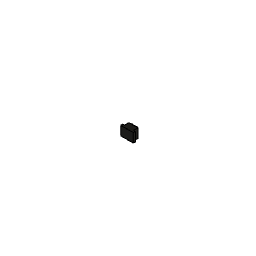
Taste7_v56 (Autodesk Fusion 360 design; units mm, degrees)
Autodesk Fusion 360 part; units mm, degrees
sketch "Skizze1" plane through (0, 0, 59.536) normal (0, 0, -1) x (1, 0, 0)
  line L0 (54.288, -85.97) -> (62.288, -85.97)
  line L1 (62.288, -85.97) -> (62.288, -82.97)
  line L2 (62.288, -82.97) -> (54.288, -82.97)
  line L3 (54.288, -82.97) -> (54.288, -85.97)
  line L4 (63.688, -82.82) -> (62.188, -82.82)
  line L5 (62.188, -82.82) -> (62.188, -86.47)
  line L6 (62.188, -86.47) -> (54.588, -86.47)
  line L7 (54.588, -86.47) -> (54.588, -82.82)
  line L8 (54.588, -82.82) -> (53.088, -82.82)
  line L9 (53.088, -82.82) -> (53.088, -81.07)
  line L10 (53.088, -81.07) -> (63.688, -81.07)
  line L11 (63.688, -81.07) -> (63.688, -82.82)
  line L12 (-67.1, -82.97) -> (67.1, -82.97)
  line L13 (56.538, -80.97) -> (60.038, -80.97)
  line L14 (50.288, -82.97) -> (50.288, -85.97)
  point P0 (54.288, -85.97)
  point P1 (50.288, -85.97)
  dimension "d139" = 1.5
  dimension "d140" = 1.5
  dimension "d1183" = 1.75
  dimension "d1184" = 3.65
  dimension "d1185" = 7.6
  constraint horizontal L4
  constraint perpendicular L0 L5
  constraint perpendicular L5 L6
  constraint perpendicular L0 L7
  constraint perpendicular L7 L8
  constraint perpendicular L0 L9
  constraint perpendicular L7 L10
  constraint perpendicular L10 L11
  constraint horizontal L4.end L7.end
  measures "d139" distance of L7.end L8.end
  measures "d140" distance of L4.start L4.end
  measures "d1183" distance of L8.end L9.end
  measures "d1184" distance of L6.end L7.end
  measures "d1185" distance of L5.end L6.end
extrude "Extrusion1" add sketch "Skizze1" along normal blind 7.6 contours L0 L2 L5 L7 L12 | L0 L5 L6 L7 | L2 L4 L5 L7 L8 L9 L10 L11 L12
sketch "Skizze2" plane through (0, 86.47, 0) normal (0, 1, 0) x (-1, 0, 0)
  line L0 (-54.588, 59.536) -> (-62.188, 59.536)
  line L1 (-62.188, 59.536) -> (-62.188, 51.936)
  line L2 (-62.188, 51.936) -> (-54.588, 51.936)
  line L3 (-54.588, 51.936) -> (-54.588, 59.536)
  line L4 (-60.8264, 52.636) -> (-55.9496, 52.636) construction
  line L5 (-55.9496, 52.636) -> (-55.9496, 61.236) construction
  line L6 (-55.9496, 61.236) -> (-60.8264, 61.236) construction
  line L7 (-60.8264, 61.236) -> (-60.8264, 52.636) construction
  point P0 (-58.388, 61.236)
  point P1 (-58.388, 59.536)
  dimension "d151" = 0.7
  dimension "d383" = 1.7
  text T0 "7" font "Arial Black" height 8.6 bold align ink ink in box 0 x 0 at (-60.8264, 52.636) x (1, 0) y (0, 1) spacing 1 height is em
  constraint perpendicular L4 L5
  constraint parallel L4 L6
  constraint parallel L5 L7
  constraint midpoint L6 P0
  constraint midpoint L0 P1
  constraint vertical P0 P1
  measures "d151" distance of L2 L4
  measures "d383" distance of L0 L6
emboss "Prägen1" depth 1 profiles "Skizze2" section 1 text T0 onto face at (59.6547, 86.47, 54.4693)
move_body "Verschieben1" bodies 1 to x (1, 0, 0) y (0, 1, 0) z (0, 0, 1) at (0, 0, 0.2)
equation "d140 = d139"
